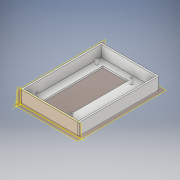
# Autodesk Inventor part: receiver-box
Saved by Autodesk Inventor 2017 (Build 210142000, 142)
## iProperties
Created: 2020-06-15
Part Number: receiver-box
Material: ABS Plastic
Document SubType Name: Modeling
Designer: HAYNIE
Density: 1.06 g/cm^3
Appearance: Smooth - White
Author: HAYNIE
Autodesk Inventor part; units mm, degrees
sketch "Box-Sketch" plane through (0, 0, 0) normal (0, 1, 0) x (-1, 0, 0)
  line L0 (23.8408, 12.5176) -> (-66.1592, 12.5176)
  line L1 (-66.1592, 12.5176) -> (-66.1592, -112.4824)
  line L2 (-66.1592, -112.4824) -> (23.8408, -112.4824)
  line L3 (23.8408, -112.4824) -> (23.8408, 12.5176)
  point P0 (0, 0)
  dimension "d0" = 90
  dimension "d1" = 125
  constraints: 8 end point, 2 parallel, 1 horizontal, 1 perpendicular
  measures "d0" distance of L2.end L1.end
  measures "d1" distance of L1.end L0.end
extrude "Box-Extrude" add sketch "Box-Sketch" along normal blind 20
shell "Box-Shell" thickness 2.54 removed faces 1 at (6.1592, 20, -70.8157)
sketch "LCD-Sketch" plane through (-21.3008, 2.54, 9.9776) normal (0, 1, 0) x (1, 0, 0)
  line L0 (12.6293, 12.7312) -> (52.1293, 12.7312)
  line L1 (52.1293, 12.7312) -> (52.1293, 109.7312)
  line L2 (52.1293, 109.7312) -> (12.6293, 109.7312)
  line L3 (12.6293, 109.7312) -> (12.6293, 12.7312)
  point P0 (21.3008, 9.9776)
  dimension "d41" = 39.5
  dimension "d42" = 97
  constraints: 8 end point, 2 parallel, 1 horizontal, 1 perpendicular
  measures "d41" distance of L2.end L1.end
  measures "d42" distance of L1.end L0.end
extrude "LCD-Extrude" cut sketch "LCD-Sketch" along normal mid plane 76.2
sketch "LCD-Posts" plane through (-21.3008, 2.54, 9.9776) normal (0, 1, 0) x (1, 0, 0)
  circle A0 centre (5.6293, 107.5979) radius 2
  circle A1 centre (59.1293, 107.7876) radius 2
  circle A2 centre (59.1293, 14.7168) radius 2
  circle A3 centre (5.632, 14.7168) radius 2
  constraints: 4 centre point
extrude "Extrusion3" add sketch "LCD-Posts" along normal blind 8
hole "Hole6" at (-15.7162, 10.54, -4.6343) direction (0, -1, 0) diameter 1.5 depth 5
hole "Hole7" at (-15.6506, 10.54, -97.6308) direction (0, -1, 0) diameter 1.5 depth 5
hole "Hole8" at (37.8285, 10.54, -97.8205) direction (0, -1, 0) diameter 1.5 depth 5
hole "Hole9" at (37.8494, 10.54, -4.7497) direction (0, -1, 0) diameter 1.5 depth 5
fillet "Fillet1" radius 2 1 edges at (21.1592, 0, -112.4824)
fillet "Fillet2" radius 2 3 edges at (-23.8408, 0, -48.9824) (-23.8408, 0.5858, -111.8966) (-23.8408, 11, -112.4824)
fillet "Fillet3" radius 2 3 edges at (66.1592, 0, -48.9824) (66.1592, 0.5858, -111.8966) (66.1592, 11, -112.4824)
fillet "Fillet4" radius 2 5 edges at (21.1592, 0, 12.5176) (65.5734, 0.5858, 12.5176) (66.1592, 11, 12.5176) (-23.255, 0.5858, 12.5176) (-23.8408, 11, 12.5176)
move or copy body "Move Body1" bodies to move or copy 1 copy no translate (0, 0, -12.51)
move or copy body "Move Body2" bodies to move or copy 1 copy no translate (23.83, 0, 0)
body "Solid1"
